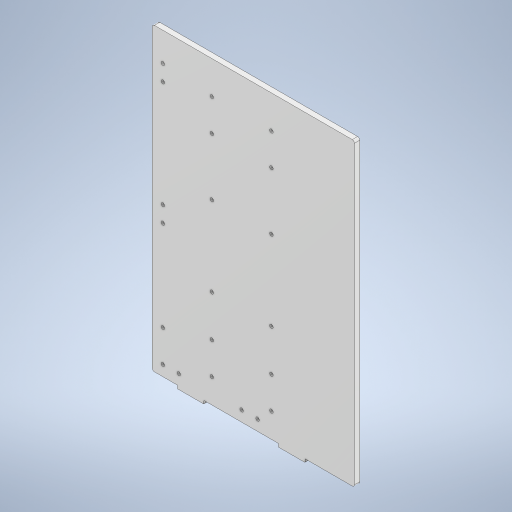
# Autodesk Inventor part: BP_Exterior-Right-Ver2
Saved by Autodesk Inventor 2024.3 (Build 283343000, 343)
## iProperties
Created: 2025-04-22
Part Number: BP_Exterior-Right-Ver2
Material: PBT プラスチック
Document SubType Name: Modeling
Designer: ngt-a
Density: 1.31 g/cm^3
Appearance: 滑らか - 白
Mass: 278.324 g
Surface Area: 1185.79 cm^2
Volume: 212.461 cm^3
Author: ngt-a
Autodesk Inventor part; units mm, degrees
ref_plane "YZ Plane" through (0, 0, 0) normal (1, 0, 0) x (0, 1, 0)
ref_plane "XZ Plane" through (0, 0, 0) normal (0, 1, 0) x (-1, 0, 0)
ref_plane "XY Plane" through (0, 0, 0) normal (0, 0, 1) x (1, 0, 0)
sketch "スケッチ22" plane through (0, 0, 0) normal (0, 0, 1) x (1, 0, 0)
  line L0 (0, 0) -> (190, 0)
  line L1 (190, 0) -> (190, 305)
  line L2 (190, 305) -> (0, 305)
  line L3 (0, 305) -> (0, 0)
  dimension "d163" = 190
  dimension "d164" = 305
  constraints: 8 end point, 2 parallel, 1 horizontal, 1 perpendicular
  measures "d163" distance of L1.end L2.end
  measures "d164" distance of L0.end L1.end
extrude "押し出し20" add sketch "スケッチ22" along normal blind 3
sketch "スケッチ23" plane through (0, 0, 3) normal (0, 0, 1) x (1, 0, 0)
  line L0 (0, 0) -> (190, 0) projected
  line L1 (190, 0) -> (190, 305) projected
  line L2 (0, 305) -> (0, 0) projected
  line L3 (190, 305) -> (0, 305) projected
  point P0 (134, 26)
  point P1 (78, 26)
  point P2 (78, 56)
  point P3 (134, 56)
  point P4 (78, 224)
  point P5 (134, 224)
  point P6 (134, 254)
  point P7 (78, 254)
  point P8 (134, 95)
  point P9 (134, 170)
  point P10 (78, 170)
  point P11 (78, 95)
  dimension "d167" = 56
  dimension "d168" = 30
  dimension "d169" = 30
  dimension "d170" = 56
  dimension "d171" = 56
  dimension "d172" = 56
  dimension "d173" = 30
  dimension "d174" = 30
  dimension "d175" = 75
  dimension "d176" = 75
  dimension "d177" = 56
  dimension "d178" = 56
  dimension "d179" = 26
  dimension "d180" = 26
  dimension "d181" = 39
  dimension "d182" = 39
  dimension "d183" = 54
  dimension "d184" = 54
  dimension "d185" = 56
  dimension "d316" = 56
  dimension "d317" = 56
  dimension "d318" = 78
  dimension "d319" = 51
  measures "d167" distance of point (134, 56) point (78, 56)
  measures "d168" distance of point (134, 26) point (134, 56)
  measures "d169" distance of point (78, 56) point (78, 26)
  measures "d170" distance of point (134, 26) point (78, 26)
  measures "d171" distance of point (134, 224) point (78, 224)
  measures "d172" distance of point (134, 254) point (78, 254)
  measures "d173" distance of point (134, 224) point (134, 254)
  measures "d174" distance of point (78, 254) point (78, 224)
  measures "d175" distance of point (134, 95) point (134, 170)
  measures "d176" distance of point (78, 170) point (78, 95)
  measures "d177" distance of point (134, 95) point (78, 95)
  measures "d178" distance of point (134, 170) point (78, 170)
  measures "d179" distance from line of L0 point (134, 26)
  measures "d180" distance from line of L0 point (78, 26)
  measures "d181" distance of point (134, 56) point (134, 95)
  measures "d182" distance of point (78, 56) point (78, 95)
  measures "d183" distance of point (134, 170) point (134, 224)
  measures "d184" distance of point (78, 170) point (78, 224)
  measures "d185" distance from line of L1 point (134, 26)
  measures "d316" distance from line of L1 point (134, 224)
  measures "d317" distance from line of L1 point (134, 254)
  measures "d318" distance from line of L2 point (78, 254)
  measures "d319" distance from line of L3 point (78, 254)
hole "穴2" at (134, 26, 3) at (78, 26, 3) at (78, 56, 3) at (134, 56, 3) at (78, 224, 3) at (134, 224, 3) at (134, 254, 3) at (78, 254, 3) at (134, 95, 3) at (134, 170, 3) at (78, 170, 3) at (78, 95, 3) direction (0, 0, -1) diameter 3.2 end through all
sketch "スケッチ24" plane through (0, 0, 3) normal (0, 0, 1) x (1, 0, 0)
  line L0 (0, 305) -> (0, 0) projected
  line L1 (0, 0) -> (190, 0) projected
  line L2 (190, 0) -> (190, 305) projected
  point P0 (91, 13)
  point P1 (106, 13)
  point P2 (165, 13)
  point P3 (180, 13)
  dimension "d193" = 15
  dimension "d195" = 13
  dimension "d196" = 13
  dimension "d204" = 15
  dimension "d205" = 13
  dimension "d207" = 13
  dimension "d217" = 59
  dimension "d219" = 10
  measures "d193" distance of point (106, 13) point (91, 13)
  measures "d195" distance from line of L1 point (106, 13)
  measures "d196" distance from line of L1 point (91, 13)
  measures "d204" distance of point (165, 13) point (180, 13)
  measures "d205" distance from line of L1 point (165, 13)
  measures "d207" distance from line of L1 point (180, 13)
  measures "d217" distance of point (106, 13) point (165, 13)
  measures "d219" distance from line of L2 point (180, 13)
hole "穴3" at (91, 13, 3) at (106, 13, 3) at (165, 13, 3) at (180, 13, 3) direction (0, 0, -1) diameter 3.2 end through all
sketch "スケッチ25" plane through (0, 0, 3) normal (0, 0, 1) x (1, 0, 0)
  line L0 (0, 0) -> (46.3, 0)
  line L1 (46.3, 0) -> (46.3, 3)
  line L2 (46.3, 3) -> (0, 3)
  line L3 (0, 3) -> (0, 0)
  line L4 (71.5, 0) -> (141.3, 0)
  line L5 (141.3, 0) -> (141.3, 3)
  line L6 (141.3, 3) -> (71.5, 3)
  line L7 (71.5, 3) -> (71.5, 0)
  line L8 (190, 0) -> (190, 305) projected
  line L9 (190, 0) -> (166.5, 0)
  line L10 (166.5, 0) -> (166.5, 3)
  line L11 (166.5, 3) -> (190, 3)
  line L12 (190, 3) -> (190, 0)
  point P0 (46.3, 1.5)
  point P1 (71.5, 1.5)
  point P2 (166.5, 1.5)
  point P3 (141.3, 1.5)
  point P4 (190, 1.5)
  dimension "d209" = 3
  dimension "d210" = 3
  dimension "d211" = 3
  dimension "d212" = 25.2
  dimension "d213" = 25.2
  dimension "d221" = 23.5
  dimension "d222" = 69.8
  constraints: 24 end point, 6 parallel, 5 midpoint, 3 horizontal, 3 perpendicular, 1 point on line
  measures "d209" distance of L0.end L1.end
  measures "d210" distance between parallel lines of L4 L6
  measures "d211" distance between parallel lines of L9 L11
  measures "d212" distance of point (46.3, 1.5) point (71.5, 1.5)
  measures "d213" distance of point (166.5, 1.5) point (141.3, 1.5)
  measures "d221" distance of point (190, 1.5) point (166.5, 1.5)
  measures "d222" distance of L5.end L6.end
extrude "押し出し21" cut sketch "スケッチ25" against normal through all
sketch "スケッチ26" plane through (0, 0, 0) normal (0, 0, -1) x (-1, 0, 0)
  line L0 (-190, 305) -> (0, 305) projected
  line L1 (0, 305) -> (0, 3) projected
  line L2 (-190, 305) -> (0, 305)
  line L3 (0, 305) -> (0, 285)
  line L4 (0, 285) -> (-190, 285)
  line L5 (-190, 285) -> (-190, 305)
  line L6 (0, 305) -> (-10, 305)
  line L7 (-10, 305) -> (-10, 0)
  line L8 (-10, 0) -> (0, 0)
  line L9 (0, 0) -> (0, 305)
  line L10 (-141.3, 0) -> (-166.5, 0) projected
  line L11 (-190, 3) -> (-190, 305) projected
  point P0 (0, 0)
  point P1 (-10, 285)
  dimension "d223" = 20
  dimension "d228" = 305
  dimension "d229" = 190
  constraints: 16 end point, 4 parallel, 2 horizontal, 2 perpendicular, 1 point on line
  measures "d223" distance between parallel lines of L0 L4
  measures "d228" distance between parallel lines of L10 L0
  measures "d229" distance between parallel lines of L1 L11
extrude "押し出し22" cut sketch "スケッチ26" against normal blind 10 contours L0 L7 L4 L5 | L0 L1 L4 L7
fillet "フィレット2" radius 2 4 edges at (190, 285, 1.5) (190, 3, 1.5) (0, 3, 1.5) (0, 285, 1.5)
sketch "スケッチ27" plane through (141.3, 0, 0) normal (0, -1, 0) x (1, 0, 0)
  line L0 (-95, 3) -> (-69.8, 3) projected
  line L1 (-69.8, 3) -> (-95, 3)
  line L2 (-95, 3) -> (-95, 0)
  line L3 (-95, 0) -> (-69.8, 0)
  line L4 (-69.8, 0) -> (-69.8, 3)
  line L5 (25.2, 3) -> (25.2, 0) projected
  line L6 (25.2, 3) -> (0, 3)
  line L7 (0, 3) -> (0, 0)
  line L8 (0, 0) -> (25.2, 0)
  line L9 (25.2, 0) -> (25.2, 3)
  line L10 (-69.9, 0.1) -> (-94.9, 0.1)
  line L11 (-94.9, 0.1) -> (-94.9, 2.9)
  line L12 (-94.9, 2.9) -> (-69.9, 2.9)
  line L13 (-69.9, 2.9) -> (-69.9, 0.1)
  line L14 (25.1, 0.1) -> (0.1, 0.1)
  line L15 (0.1, 0.1) -> (0.1, 2.9)
  line L16 (0.1, 2.9) -> (25.1, 2.9)
  line L17 (25.1, 2.9) -> (25.1, 0.1)
  line L18 (-69.8, 3) -> (-69.9, 3)
  line L19 (-69.9, 3) -> (-69.9, 0)
  line L20 (-69.9, 0) -> (-69.8, 0)
  line L21 (-69.8, 0) -> (-69.8, 3)
  line L22 (-95, 3) -> (-94.9, 3)
  line L23 (-94.9, 3) -> (-94.9, 0)
  line L24 (-94.9, 0) -> (-95, 0)
  line L25 (-95, 0) -> (-95, 3)
  line L26 (0, 3) -> (0.1, 3)
  line L27 (0.1, 3) -> (0.1, 0)
  line L28 (0.1, 0) -> (0, 0)
  line L29 (0, 0) -> (0, 3)
  line L30 (25.2, 3) -> (25.1, 3)
  line L31 (25.1, 3) -> (25.1, 0)
  line L32 (25.1, 0) -> (25.2, 0)
  line L33 (25.2, 0) -> (25.2, 3)
  point P0 (-141.3, 0)
  point P1 (-69.8, 1.5)
  point P2 (-95, 1.5)
  point P3 (0.1, 2.9)
  point P4 (0.1, 3)
  point P5 (0.1, 0.1)
  point P6 (25.1, 0.1)
  point P7 (25.1, 3)
  point P8 (25.1, 2.9)
  dimension "d231" = 3
  dimension "d232" = 25.2
  dimension "d233" = 0.1
  dimension "d234" = 0.1
  constraints: 64 end point, 16 parallel, 8 perpendicular, 6 horizontal, 6 point on line, 2 midpoint, 6 other
  measures "d231" distance between parallel lines of L0 L3
  measures "d232" distance of point (-69.8, 1.5) point (-95, 1.5)
  measures "d233" distance between parallel lines of L8 L14
  measures "d234" distance between parallel lines of L3 L10
extrude "押し出し23" cut sketch "スケッチ27" against normal blind 3 contours L0 L23 L11 L3 L2 | L0 L4 L3 L19 L13 | L5 L8 L31 L17 L6 | L27 L15 L8 L7 L6
sketch "スケッチ28" plane through (0, 0, 0) normal (0, 0, -1) x (-1, 0, 0)
  line L0 (-71.4, 3) -> (-71.4, 0) projected
  line L1 (-46.4, 0) -> (-71.4, 0) projected
  line L2 (-46.4, 0) -> (-46.4, 3) projected
  line L3 (-46.4, 3) -> (-2, 3) projected
  arc A0 (-2, 3) -> (0, 5) centre (-2, 5) ccw projected
  line L4 (0, 283) -> (0, 5) projected
  arc A1 (0, 283) -> (-2, 285) centre (-2, 283) ccw projected
  line L5 (-2, 285) -> (-188, 285) projected
  arc A2 (-188, 285) -> (-190, 283) centre (-188, 283) ccw projected
  line L6 (-190, 5) -> (-190, 283) projected
  arc A3 (-190, 5) -> (-188, 3) centre (-188, 5) ccw projected
  line L7 (-188, 3) -> (-166.4, 3) projected
  line L8 (-166.4, 3) -> (-166.4, 0) projected
  line L9 (-141.4, 0) -> (-166.4, 0) projected
  line L10 (-141.4, 0) -> (-141.4, 3) projected
  line L11 (-141.4, 3) -> (-71.4, 3) projected
  circle A4 centre (-134, 26) radius 1.6 projected
  circle A5 centre (-78, 26) radius 1.6 projected
  circle A6 centre (-78, 56) radius 1.6 projected
  circle A7 centre (-134, 56) radius 1.6 projected
  circle A8 centre (-78, 224) radius 1.6 projected
  circle A9 centre (-134, 224) radius 1.6 projected
  circle A10 centre (-134, 254) radius 1.6 projected
  circle A11 centre (-78, 254) radius 1.6 projected
  circle A12 centre (-134, 95) radius 1.6 projected
  circle A13 centre (-134, 170) radius 1.6 projected
  circle A14 centre (-78, 170) radius 1.6 projected
  circle A15 centre (-78, 95) radius 1.6 projected
  circle A16 centre (-91, 13) radius 1.6 projected
  circle A17 centre (-106, 13) radius 1.6 projected
  circle A18 centre (-165, 13) radius 1.6 projected
  circle A19 centre (-180, 13) radius 1.6 projected
  line L12 (-190, 285) -> (0, 285)
  line L13 (0, 285) -> (0, 3)
  line L14 (0, 3) -> (-190, 3)
  line L15 (-190, 3) -> (-190, 285)
  point P0 (0, 0)
  constraints: 8 end point, 2 parallel, 2 point on line, 1 horizontal, 1 perpendicular
extrude "押し出し24" add sketch "スケッチ28" along normal blind 2 contours L11 L14 L7 A3 L6 A2 L5 A1 L4 A0 L3
sketch "スケッチ29" plane through (0, 0, -2) normal (0, 0, -1) x (-1, 0, 0)
  line L0 (-188, 3) -> (-2, 3) projected
  arc A0 (-2, 3) -> (0, 5) centre (-2, 5) ccw projected
  line L1 (0, 5) -> (0, 283) projected
  arc A1 (0, 283) -> (-2, 285) centre (-2, 283) ccw projected
  line L2 (-2, 285) -> (-188, 285) projected
  arc A2 (-188, 285) -> (-190, 283) centre (-188, 283) ccw projected
  line L3 (-190, 283) -> (-190, 5) projected
  arc A3 (-190, 5) -> (-188, 3) centre (-188, 5) ccw projected
  circle A4 centre (-165, 13) radius 1.6 projected
  circle A5 centre (-91, 13) radius 1.6 projected
  circle A6 centre (-78, 170) radius 1.6 projected
  circle A7 centre (-134, 95) radius 1.6 projected
  circle A8 centre (-134, 254) radius 1.6 projected
  circle A9 centre (-134, 26) radius 1.6 projected
  circle A10 centre (-78, 26) radius 1.6 projected
  circle A11 centre (-78, 56) radius 1.6 projected
  circle A12 centre (-134, 56) radius 1.6 projected
  circle A13 centre (-78, 224) radius 1.6 projected
  circle A14 centre (-134, 224) radius 1.6 projected
  circle A15 centre (-78, 254) radius 1.6 projected
  circle A16 centre (-134, 170) radius 1.6 projected
  circle A17 centre (-78, 95) radius 1.6 projected
  circle A18 centre (-106, 13) radius 1.6 projected
  circle A19 centre (-180, 13) radius 1.6 projected
  line L4 (-190, 20) -> (0, 20)
  line L5 (-46.4, 0) -> (-71.4, 0) projected
  circle A20 centre (-134, 26) radius 3.75
  circle A21 centre (-78, 26) radius 3.75
  circle A22 centre (-134, 56) radius 3.75
  circle A23 centre (-78, 56) radius 3.75
  circle A24 centre (-134, 95) radius 3.75
  circle A25 centre (-78, 95) radius 3.75
  circle A26 centre (-134, 170) radius 3.75
  circle A27 centre (-78, 170) radius 3.75
  circle A28 centre (-134, 224) radius 3.75
  circle A29 centre (-78, 224) radius 3.75
  circle A30 centre (-134, 254) radius 3.75
  circle A31 centre (-78, 254) radius 3.75
  line L6 (-20, 285) -> (-20, 3)
  line L7 (-111.1, 20) -> (-85.9, 20)
  line L8 (-85.9, 20) -> (-85.9, 30)
  line L9 (-85.9, 30) -> (-111.1, 30)
  line L10 (-111.1, 30) -> (-111.1, 20)
  line L11 (-159.9, 20) -> (-185.1, 20)
  line L12 (-185.1, 20) -> (-185.1, 30)
  line L13 (-185.1, 30) -> (-159.9, 30)
  line L14 (-159.9, 30) -> (-159.9, 20)
  point P0 (0, 0)
  point P1 (-185.1, 25)
  point P2 (-98.5, 30)
  point P3 (-111.1, 25)
  point P4 (-20, 20)
  point P5 (-85.9, 20)
  dimension "d239" = 20
  dimension "d242" = 7.5
  dimension "d243" = 7.5
  dimension "d244" = 7.5
  dimension "d245" = 7.5
  dimension "d246" = 7.5
  dimension "d247" = 7.5
  dimension "d248" = 7.5
  dimension "d249" = 7.5
  dimension "d250" = 7.5
  dimension "d251" = 7.5
  dimension "d252" = 7.5
  dimension "d253" = 7.5
  dimension "d254" = 20
  dimension "d256" = 5.1
  dimension "d257" = 10
  dimension "d258" = 10
  dimension "d259" = 5.1
  dimension "d263" = 5.1
  dimension "d264" = 5.1
  constraints: 20 end point, 12 centre point, 6 point on line, 4 parallel, 4 perpendicular, 3 midpoint, 2 horizontal
  measures "d239" distance between parallel lines of L5 L4
  measures "d242" diameter of A30
  measures "d243" diameter of A31
  measures "d244" diameter of A28
  measures "d245" diameter of A29
  measures "d246" diameter of A26
  measures "d247" diameter of A27
  measures "d248" diameter of A24
  measures "d249" diameter of A25
  measures "d250" diameter of A22
  measures "d251" diameter of A23
  measures "d252" diameter of A20
  measures "d253" diameter of A21
  measures "d254" distance between parallel lines of L1 L6
  measures "d256" horizontal distance of A19.centre point (-185.1, 25)
  measures "d257" distance between parallel lines of L4 L13
  measures "d258" distance from line of L7 point (-98.5, 30)
  measures "d259" distance from line of A18.centre L10
  measures "d263" distance from line of A4.centre L14
  measures "d264" distance from line of A5.centre L8
extrude "押し出し25" cut sketch "スケッチ29" against normal blind 2 contours A3 L3 L4 L6 L0 | L4 L10 L9 L8 | L12 L13 L14 L4 | A6 | A7 | A8 | A9 | A12 | A13 | A14 | A15 | A16 | A17 | A20 | A21 | A22 | A23 | A24 | A25 | A26 | A27 | A28 | A29 | A30 | A31
fillet "フィレット3" radius 2 11 edges at (190, 20, -1) (185.1, 20, -1) (185.1, 30, -1) (159.9, 30, -1) (159.9, 20, -1) (111.1, 20, -1) (111.1, 30, -1) (85.9, 30, -1) (85.9, 20, -1) (20, 20, -1) (20, 3, -1)
fillet "フィレット4" radius 0.2 8 edges at (166.4, 3, 1.5) (166.4, 0, 1.5) (141.4, 0, 1.5) (141.4, 3, 1.5) (71.4, 0, 1.5) (46.4, 0, 1.5) (46.4, 3, 1.5) (71.4, 3, 1.5)
sketch "スケッチ31" plane through (0, 0, -2) normal (0, 0, -1) x (-1, 0, 0)
  circle A0 centre (-180, 13) radius 1.6 projected
  line L0 (-190, 283) -> (-190, 22) projected
  point P0 (0, 0)
  point P1 (-180, 43)
  point P2 (-180, 128)
  point P3 (-180, 258)
  point P4 (-180, 143)
  point P5 (-180, 243)
  dimension "d265" = 30
  dimension "d266" = 10
  dimension "d267" = 10
  dimension "d268" = 85
  dimension "d269" = 15
  dimension "d270" = 100
  dimension "d271" = 15
  dimension "d272" = 10
  dimension "d273" = 10
  dimension "d274" = 10
  measures "d265" distance of A0.centre point (-180, 43)
  measures "d266" distance from line of L0 point (-180, 43)
  measures "d267" distance from line of L0 point (-180, 128)
  measures "d268" distance of point (-180, 43) point (-180, 128)
  measures "d269" distance of point (-180, 128) point (-180, 143)
  measures "d270" distance of point (-180, 143) point (-180, 243)
  measures "d271" distance of point (-180, 243) point (-180, 258)
  measures "d272" distance from line of L0 point (-180, 143)
  measures "d273" distance from line of L0 point (-180, 243)
  measures "d274" distance from line of L0 point (-180, 258)
hole "穴4" at (180, 43, -2) at (180, 128, -2) at (180, 258, -2) at (180, 143, -2) at (180, 243, -2) direction (0, 0, 1) diameter 3.2 depth 61.5 tip angle 118
sketch "スケッチ32" plane through (0, 0, -2) normal (0, 0, -1) x (-1, 0, 0)
  arc A0 (-46.6, 0) -> (-46.4, 0.2) centre (-46.6, 0.2) ccw projected
  line L0 (-46.4, 0.2) -> (-46.4, 2.8) projected
  arc A1 (-46.2, 3) -> (-46.4, 2.8) centre (-46.2, 2.8) ccw projected
  line L1 (-18, 3) -> (-46.2, 3) projected
  arc A2 (-20, 5) -> (-18, 3) centre (-18, 5) ccw projected
  line L2 (-20, 18) -> (-20, 5) projected
  arc A3 (-20, 18) -> (-22, 20) centre (-22, 18) ccw projected
  line L3 (-83.9, 20) -> (-22, 20) projected
  arc A4 (-85.9, 22) -> (-83.9, 20) centre (-83.9, 22) ccw projected
  line L4 (-85.9, 28) -> (-85.9, 22) projected
  arc A5 (-85.9, 28) -> (-87.9, 30) centre (-87.9, 28) ccw projected
  line L5 (-109.1, 30) -> (-87.9, 30) projected
  arc A6 (-109.1, 30) -> (-111.1, 28) centre (-109.1, 28) ccw projected
  line L6 (-111.1, 22) -> (-111.1, 28) projected
  arc A7 (-113.1, 20) -> (-111.1, 22) centre (-113.1, 22) ccw projected
  line L7 (-157.9, 20) -> (-113.1, 20) projected
  arc A8 (-159.9, 22) -> (-157.9, 20) centre (-157.9, 22) ccw projected
  line L8 (-159.9, 28) -> (-159.9, 22) projected
  arc A9 (-159.9, 28) -> (-161.9, 30) centre (-161.9, 28) ccw projected
  line L9 (-183.1, 30) -> (-161.9, 30) projected
  arc A10 (-183.1, 30) -> (-185.1, 28) centre (-183.1, 28) ccw projected
  line L10 (-185.1, 22) -> (-185.1, 28) projected
  arc A11 (-187.1, 20) -> (-185.1, 22) centre (-187.1, 22) ccw projected
  line L11 (-188, 20) -> (-187.1, 20) projected
  arc A12 (-190, 22) -> (-188, 20) centre (-188, 22) ccw projected
  line L12 (-190, 5) -> (-190, 22) projected
  arc A13 (-190, 5) -> (-188, 3) centre (-188, 5) ccw projected
  line L13 (-166.6, 3) -> (-188, 3) projected
  arc A14 (-166.4, 2.8) -> (-166.6, 3) centre (-166.6, 2.8) ccw projected
  line L14 (-166.4, 2.8) -> (-166.4, 0.2) projected
  arc A15 (-166.4, 0.2) -> (-166.2, 0) centre (-166.2, 0.2) ccw projected
  line L15 (-141.6, 0) -> (-166.2, 0) projected
  arc A16 (-141.6, 0) -> (-141.4, 0.2) centre (-141.6, 0.2) ccw projected
  line L16 (-141.4, 0.2) -> (-141.4, 2.8) projected
  arc A17 (-141.2, 3) -> (-141.4, 2.8) centre (-141.2, 2.8) ccw projected
  line L17 (-71.6, 3) -> (-141.2, 3) projected
  arc A18 (-71.4, 2.8) -> (-71.6, 3) centre (-71.6, 2.8) ccw projected
  line L18 (-71.4, 2.8) -> (-71.4, 0.2) projected
  arc A19 (-71.4, 0.2) -> (-71.2, 0) centre (-71.2, 0.2) ccw projected
  line L19 (-46.6, 0) -> (-71.2, 0) projected
  circle A20 centre (-180, 13) radius 1.6 projected
  circle A21 centre (-106, 13) radius 1.6 projected
  circle A22 centre (-91, 13) radius 1.6 projected
  circle A23 centre (-165, 13) radius 1.6 projected
  circle A24 centre (-180, 243) radius 1.6 projected
  circle A25 centre (-180, 143) radius 1.6 projected
  circle A26 centre (-180, 258) radius 1.6 projected
  circle A27 centre (-180, 128) radius 1.6 projected
  arc A28 (-20, 5) -> (-18, 3) centre (-18, 5) ccw projected
  line L20 (-18, 3) -> (-2, 3) projected
  arc A29 (-2, 3) -> (0, 5) centre (-2, 5) ccw projected
  line L21 (0, 5) -> (0, 283) projected
  arc A30 (0, 283) -> (-2, 285) centre (-2, 283) ccw projected
  line L22 (-2, 285) -> (-188, 285) projected
  arc A31 (-188, 285) -> (-190, 283) centre (-188, 283) ccw projected
  line L23 (-190, 283) -> (-190, 22) projected
  arc A32 (-190, 22) -> (-188, 20) centre (-188, 22) ccw projected
  line L24 (-188, 20) -> (-187.1, 20) projected
  arc A33 (-187.1, 20) -> (-185.1, 22) centre (-187.1, 22) ccw projected
  line L25 (-185.1, 22) -> (-185.1, 28) projected
  arc A34 (-183.1, 30) -> (-185.1, 28) centre (-183.1, 28) ccw projected
  line L26 (-183.1, 30) -> (-161.9, 30) projected
  arc A35 (-159.9, 28) -> (-161.9, 30) centre (-161.9, 28) ccw projected
  line L27 (-159.9, 28) -> (-159.9, 22) projected
  arc A36 (-159.9, 22) -> (-157.9, 20) centre (-157.9, 22) ccw projected
  line L28 (-157.9, 20) -> (-113.1, 20) projected
  arc A37 (-113.1, 20) -> (-111.1, 22) centre (-113.1, 22) ccw projected
  line L29 (-111.1, 22) -> (-111.1, 28) projected
  arc A38 (-109.1, 30) -> (-111.1, 28) centre (-109.1, 28) ccw projected
  line L30 (-109.1, 30) -> (-87.9, 30) projected
  arc A39 (-85.9, 28) -> (-87.9, 30) centre (-87.9, 28) ccw projected
  line L31 (-85.9, 28) -> (-85.9, 22) projected
  arc A40 (-85.9, 22) -> (-83.9, 20) centre (-83.9, 22) ccw projected
  line L32 (-83.9, 20) -> (-22, 20) projected
  arc A41 (-20, 18) -> (-22, 20) centre (-22, 18) ccw projected
  line L33 (-20, 18) -> (-20, 5) projected
  circle A42 centre (-78, 26) radius 3.75 projected
  circle A43 centre (-78, 170) radius 3.75 projected
  circle A44 centre (-78, 254) radius 3.75 projected
  circle A45 centre (-134, 224) radius 3.75 projected
  circle A46 centre (-134, 95) radius 3.75 projected
  circle A47 centre (-134, 26) radius 3.75 projected
  circle A48 centre (-78, 56) radius 3.75 projected
  circle A49 centre (-134, 170) radius 3.75 projected
  circle A50 centre (-134, 254) radius 3.75 projected
  circle A51 centre (-78, 224) radius 3.75 projected
  circle A52 centre (-78, 95) radius 3.75 projected
  circle A53 centre (-134, 56) radius 3.75 projected
  circle A54 centre (-180, 128) radius 3.75
  circle A55 centre (-180, 143) radius 3.75
  circle A56 centre (-180, 243) radius 3.75
  circle A57 centre (-180, 258) radius 3.75
  circle A58 centre (-180, 243) radius 1.6 projected
  circle A59 centre (-180, 143) radius 1.6 projected
  circle A60 centre (-180, 258) radius 1.6 projected
  circle A61 centre (-180, 128) radius 1.6 projected
  circle A62 centre (-180, 43) radius 1.6 projected
  arc A63 (-20, 5) -> (-18, 3) centre (-18, 5) ccw projected
  line L34 (-18, 3) -> (-2, 3) projected
  arc A64 (-2, 3) -> (0, 5) centre (-2, 5) ccw projected
  line L35 (0, 5) -> (0, 283) projected
  arc A65 (0, 283) -> (-2, 285) centre (-2, 283) ccw projected
  line L36 (-2, 285) -> (-188, 285) projected
  arc A66 (-188, 285) -> (-190, 283) centre (-188, 283) ccw projected
  line L37 (-190, 283) -> (-190, 22) projected
  arc A67 (-190, 22) -> (-188, 20) centre (-188, 22) ccw projected
  line L38 (-188, 20) -> (-187.1, 20) projected
  arc A68 (-187.1, 20) -> (-185.1, 22) centre (-187.1, 22) ccw projected
  line L39 (-185.1, 22) -> (-185.1, 28) projected
  arc A69 (-183.1, 30) -> (-185.1, 28) centre (-183.1, 28) ccw projected
  line L40 (-183.1, 30) -> (-161.9, 30) projected
  arc A70 (-159.9, 28) -> (-161.9, 30) centre (-161.9, 28) ccw projected
  line L41 (-159.9, 28) -> (-159.9, 22) projected
  arc A71 (-159.9, 22) -> (-157.9, 20) centre (-157.9, 22) ccw projected
  line L42 (-157.9, 20) -> (-113.1, 20) projected
  arc A72 (-113.1, 20) -> (-111.1, 22) centre (-113.1, 22) ccw projected
  line L43 (-111.1, 22) -> (-111.1, 28) projected
  arc A73 (-109.1, 30) -> (-111.1, 28) centre (-109.1, 28) ccw projected
  line L44 (-109.1, 30) -> (-87.9, 30) projected
  arc A74 (-85.9, 28) -> (-87.9, 30) centre (-87.9, 28) ccw projected
  line L45 (-85.9, 28) -> (-85.9, 22) projected
  arc A75 (-85.9, 22) -> (-83.9, 20) centre (-83.9, 22) ccw projected
  line L46 (-83.9, 20) -> (-22, 20) projected
  arc A76 (-20, 18) -> (-22, 20) centre (-22, 18) ccw projected
  line L47 (-20, 18) -> (-20, 5) projected
  circle A77 centre (-78, 26) radius 3.75 projected
  circle A78 centre (-78, 170) radius 3.75 projected
  circle A79 centre (-78, 254) radius 3.75 projected
  circle A80 centre (-134, 224) radius 3.75 projected
  circle A81 centre (-134, 95) radius 3.75 projected
  circle A82 centre (-134, 26) radius 3.75 projected
  circle A83 centre (-78, 56) radius 3.75 projected
  circle A84 centre (-134, 170) radius 3.75 projected
  circle A85 centre (-134, 254) radius 3.75 projected
  circle A86 centre (-78, 224) radius 3.75 projected
  circle A87 centre (-78, 95) radius 3.75 projected
  circle A88 centre (-134, 56) radius 3.75 projected
  circle A89 centre (-180, 43) radius 3.75
  point P0 (0, 0)
  dimension "d282" = 7.5
  dimension "d283" = 7.5
  dimension "d284" = 7.5
  dimension "d285" = 7.5
  dimension "d289" = 7.5
  constraints: 5 centre point
  measures "d282" diameter of A57
  measures "d283" diameter of A56
  measures "d284" diameter of A55
  measures "d285" diameter of A54
  measures "d289" diameter of A89
extrude "押し出し26" cut sketch "スケッチ32" against normal blind 2 contours A24 | A25 | A26 | A27 | A54 | A55 | A56 | A57 | A89
sketch "スケッチ34" plane through (0, 0, -2) normal (0, 0, -1) x (-1, 0, 0)
  circle A0 centre (-134, 56) radius 1.6 projected
  circle A1 centre (-78, 26) radius 1.6 projected
  line L0 (-134, 56) -> (-78, 26)
  circle A2 centre (-134, 26) radius 1.6 projected
  line L1 (-78, 26) -> (-134, 26)
  circle A3 centre (-78, 56) radius 1.6 projected
  line L2 (-134, 26) -> (-78, 56)
  line L3 (-78, 56) -> (-134, 56)
  line L4 (-134, 26) -> (-134, 56)
  line L5 (-78, 26) -> (-78, 56)
  circle A4 centre (-134, 95) radius 1.6 projected
  line L6 (-134, 95) -> (-78, 95)
  circle A5 centre (-78, 170) radius 1.6 projected
  line L7 (-78, 95) -> (-78, 170)
  circle A6 centre (-134, 170) radius 1.6 projected
  line L8 (-78, 170) -> (-134, 170)
  line L9 (-134, 170) -> (-134, 95)
  circle A7 centre (-78, 170) radius 3.75 projected
  line L10 (-78, 170) -> (-134, 95)
  line L11 (-78, 95) -> (-134, 170)
  circle A8 centre (-134, 224) radius 1.6 projected
  circle A9 centre (-134, 254) radius 1.6 projected
  line L12 (-134, 224) -> (-134, 254)
  circle A10 centre (-78, 254) radius 1.6 projected
  line L13 (-134, 254) -> (-78, 254)
  circle A11 centre (-78, 224) radius 1.6 projected
  line L14 (-78, 254) -> (-78, 224)
  line L15 (-78, 224) -> (-134, 224)
  line L16 (-78, 254) -> (-134, 224)
  line L17 (-134, 254) -> (-78, 224)
  line L18 (-134, 251) -> (-78, 251)
  line L19 (-132.5833, 256.6444) -> (-76.5833, 226.6444)
  line L20 (-79.4167, 256.6444) -> (-135.4167, 226.6444)
  line L21 (-131, 224) -> (-131, 254)
  line L22 (-135.4167, 251.3556) -> (-79.4167, 221.3556)
  line L23 (-78, 227) -> (-134, 227)
  line L24 (-76.5833, 251.3556) -> (-132.5833, 221.3556)
  line L25 (-81, 254) -> (-81, 224)
  line L26 (-134, 167) -> (-81, 167)
  line L27 (-81, 167) -> (-81, 95)
  line L28 (-131, 170) -> (-131, 95)
  line L29 (-134, 98) -> (-78, 98)
  line L30 (-75.5962, 168.2051) -> (-131.5962, 93.2051)
  line L31 (-80.4038, 93.2051) -> (-136.4038, 168.2051)
  line L32 (-80.4038, 171.7949) -> (-136.4038, 96.7949)
  line L33 (-75.5962, 96.7949) -> (-131.5962, 171.7949)
  line L34 (-78, 53) -> (-134, 53)
  line L35 (-132.5833, 58.6444) -> (-66.047, 23)
  line L36 (-66.047, 23) -> (-134, 23)
  line L37 (-81, 26) -> (-81, 56)
  line L38 (-132.5833, 23.3556) -> (-76.5833, 53.3556)
  line L39 (-135.4167, 53.3556) -> (-89.953, 29)
  line L40 (-89.953, 29) -> (-134, 29)
  line L41 (-131, 26) -> (-131, 56)
  line L42 (-135.4167, 28.6444) -> (-79.4167, 58.6444)
  circle A12 centre (-134, 224) radius 3.75 projected
  line L43 (-134, 224) -> (-134, 170)
  line L44 (-78, 224) -> (-78, 170)
  line L45 (-134, 95) -> (-134, 56)
  circle A13 centre (-78, 95) radius 1.6 projected
  line L46 (-78, 95) -> (-78, 56)
  line L47 (-134, 56) -> (-78, 95)
  line L48 (-134, 95) -> (-78, 56)
  line L49 (-134, 170) -> (-78, 224)
  line L50 (-134, 224) -> (-78, 170)
  line L51 (-78, 221) -> (-134, 221)
  line L52 (-131, 170) -> (-131, 216.9396)
  line L53 (-131, 216.9396) -> (-80.0824, 167.8405)
  line L54 (-75.9176, 172.1595) -> (-137, 231.0604)
  line L55 (-137, 231.0604) -> (-137, 170)
  line L56 (-136.0824, 172.1595) -> (-80.0824, 226.1595)
  line L57 (-131.9176, 167.8405) -> (-75.9176, 221.8405)
  line L58 (-134, 173) -> (-75, 173)
  line L59 (-75, 173) -> (-75, 95)
  line L60 (-81, 224) -> (-81, 170)
  line L61 (-134, 92) -> (-78, 92)
  line L62 (-131, 95) -> (-131, 56)
  line L63 (-81, 56) -> (-81, 89.2549)
  line L64 (-81, 89.2549) -> (-132.2855, 53.5382)
  line L65 (-132.2855, 97.4618) -> (-76.2855, 58.4618)
  line L66 (-135.7145, 58.4618) -> (-75, 100.7451)
  line L67 (-75, 100.7451) -> (-75, 56)
  line L68 (-78, 59) -> (-134, 59)
  line L69 (-135.7145, 92.5382) -> (-79.7145, 53.5382)
  point P0 (0, 0)
  point P1 (-131, 239)
  point P2 (-131, 41)
  point P3 (-81, 229.0105)
  point P4 (-81, 248.9895)
  point P5 (-99.647, 239)
  point P6 (-106, 235.5966)
  point P7 (-122.047, 227)
  point P8 (-89.953, 227)
  point P9 (-112.353, 239)
  point P10 (-131, 248.9895)
  point P11 (-131, 229.0105)
  point P12 (-106, 242.4034)
  point P13 (-89.953, 251)
  point P14 (-122.047, 251)
  point P15 (-81, 50.9895)
  point P16 (-99.647, 41)
  point P17 (-81, 31.0105)
  point P18 (-131, 31.0105)
  point P19 (-112.353, 41)
  point P20 (-131, 50.9895)
  point P21 (-106, 44.4034)
  point P22 (-89.953, 53)
  point P23 (-122.047, 53)
  point P24 (-83.984, 98)
  point P25 (-106, 127.4857)
  point P26 (-128.016, 98)
  point P27 (-128.016, 167)
  point P28 (-106, 137.5143)
  point P29 (-83.984, 167)
  point P30 (-102.256, 132.5)
  point P31 (-81, 104.0322)
  point P32 (-81, 160.9678)
  point P33 (-131, 104.0322)
  point P34 (-109.744, 132.5)
  point P35 (-131, 160.9678)
  point P36 (-100.7506, 75.5)
  point P37 (-81, 61.7451)
  point P38 (-87.5571, 59)
  point P39 (-106, 71.8442)
  point P40 (-124.4429, 59)
  point P41 (-111.2494, 75.5)
  point P42 (-131, 89.2549)
  point P43 (-131, 61.7451)
  point P44 (-106, 79.1558)
  point P45 (-87.5571, 92)
  point P46 (-124.4429, 92)
  point P47 (-81, 177.0604)
  point P48 (-81, 216.9396)
  point P49 (-101.6781, 197)
  point P50 (-126.567, 173)
  point P51 (-85.433, 173)
  point P52 (-106, 192.8324)
  point P53 (-131, 177.0604)
  point P54 (-110.3219, 197)
  point P55 (-106, 201.1676)
  point P56 (-85.433, 221)
  point P57 (-126.567, 221)
  dimension "d290" = 3
  dimension "d291" = 3
  dimension "d292" = 3
  dimension "d293" = 3
  dimension "d294" = 3
  dimension "d295" = 3
  dimension "d296" = 3
  dimension "d297" = 3
  dimension "d298" = 3
  dimension "d299" = 3
  dimension "d300" = 3
  dimension "d301" = 3
  dimension "d302" = 3
  dimension "d303" = 3
  dimension "d304" = 3
  dimension "d305" = 3
  dimension "d306" = 3
  dimension "d307" = 3
  dimension "d308" = 3
  dimension "d309" = 3
  dimension "d310" = 3
  dimension "d311" = 3
  dimension "d320" = 3
  dimension "d321" = 3
  dimension "d322" = 3
  dimension "d323" = 3
  dimension "d324" = 3
  dimension "d325" = 3
  dimension "d326" = 3
  dimension "d327" = 3
  dimension "d328" = 3
  dimension "d329" = 3
  dimension "d330" = 3
  dimension "d331" = 3
  dimension "d332" = 3
  dimension "d333" = 3
  constraints: 140 end point, 32 parallel, 9 perpendicular, 2 midpoint, 2 vertical, 1 horizontal, 1 point on line, 8 other
  measures "d290" distance between parallel lines of L13 L18
  measures "d291" distance from line of L12 point (-131, 239)
  measures "d292" distance between parallel lines of L14 L25
  measures "d293" distance between parallel lines of L15 L23
  measures "d294" distance between parallel lines of L16 L24
  measures "d295" distance between parallel lines of L20 L16
  measures "d296" distance between parallel lines of L17 L19
  measures "d297" distance between parallel lines of L17 L22
  measures "d298" distance between parallel lines of L8 L26
  measures "d299" distance between parallel lines of L9 L28
  measures "d300" distance between parallel lines of L6 L29
  measures "d301" distance between parallel lines of L10 L32
  measures "d302" distance between parallel lines of L10 L30
  measures "d303" distance between parallel lines of L11 L33
  measures "d304" distance between parallel lines of L31 L11
  measures "d305" distance between parallel lines of L3 L34
  measures "d306" distance between parallel lines of L2 L42
  measures "d307" distance between parallel lines of L38 L2
  measures "d308" distance between parallel lines of L0 L35
  measures "d309" distance between parallel lines of L39 L0
  measures "d310" distance from line of L4 point (-131, 41)
  measures "d311" distance between parallel lines of L5 L37
  measures "d320" distance between parallel lines of L15 L51
  measures "d321" distance between parallel lines of L54 L50
  measures "d322" distance between parallel lines of L53 L50
  measures "d323" distance between parallel lines of L49 L56
  measures "d324" distance between parallel lines of L57 L49
  measures "d325" distance between parallel lines of L44 L60
  measures "d326" distance between parallel lines of L8 L58
  measures "d327" distance between parallel lines of L6 L61
  measures "d328" distance between parallel lines of L48 L65
  measures "d329" distance between parallel lines of L69 L48
  measures "d330" distance between parallel lines of L45 L62
  measures "d331" distance between parallel lines of L47 L66
  measures "d332" distance between parallel lines of L47 L64
  measures "d333" distance between parallel lines of L3 L68
extrude "押し出し27" cut sketch "スケッチ34" against normal blind 2 contours L34 L42 L35 | L64 L69 L68 | L62 L69 L66 | L39 L42 L41 | L38 L37 L35 | L64 L63 L65 | L65 L61 L66 | L28 L31 L32 | L30 L31 L29 | L33 L26 L32 | L30 L27 L33 | L52 L53 L56 | L57 L53 L58 | L51 L56 L54 | L57 L60 L54 | L22 L20 L21 | L24 L22 L23 | L18 L20 L19 | L24 L25 L19
sketch "スケッチ36" plane through (0, 0, -2) normal (0, 0, -1) x (-1, 0, 0)
  line L0 (-2, 285) -> (-188, 285) projected
  line L1 (-166.5226, 285) -> (-144, 285)
  line L2 (-144, 285) -> (-144, 15.7473)
  line L3 (-144, 15.7473) -> (-166.5226, 15.7473)
  line L4 (-166.5226, 15.7473) -> (-166.5226, 285)
  line L5 (-68, 285) -> (-20, 285)
  line L6 (-20, 285) -> (-20, 11.3003)
  line L7 (-20, 11.3003) -> (-68, 11.3003)
  line L8 (-68, 11.3003) -> (-68, 285)
  line L9 (-190, 5) -> (-190, 283) projected
  line L10 (0, 285) -> (-190, 285)
  line L11 (-190, 285) -> (-190, 265)
  line L12 (-190, 265) -> (0, 265)
  line L13 (0, 265) -> (0, 285)
  line L14 (0, 5) -> (0, 283) projected
  circle A0 centre (-78, 254) radius 3.75 projected
  circle A1 centre (-134, 254) radius 3.75 projected
  line L15 (-126.567, 173) -> (-106, 192.8324) projected
  line L16 (-106, 192.8324) -> (-85.433, 173) projected
  line L17 (-85.433, 173) -> (-126.567, 173) projected
  line L18 (-87.5571, 59) -> (-124.4429, 59) projected
  line L19 (-124.4429, 59) -> (-106, 71.8442) projected
  line L20 (-106, 71.8442) -> (-87.5571, 59) projected
  line L21 (-128.016, 167) -> (-83.984, 167) projected
  line L22 (-83.984, 167) -> (-106, 137.5143) projected
  line L23 (-106, 137.5143) -> (-128.016, 167) projected
  line L24 (-81, 50.9895) -> (-81, 31.0105) projected
  line L25 (-81, 31.0105) -> (-99.647, 41) projected
  line L26 (-99.647, 41) -> (-81, 50.9895) projected
  line L27 (-81, 229.0105) -> (-99.647, 239) projected
  line L28 (-99.647, 239) -> (-81, 248.9895) projected
  line L29 (-81, 248.9895) -> (-81, 229.0105) projected
  line L30 (-106, 242.4034) -> (-122.047, 251) projected
  line L31 (-122.047, 251) -> (-89.953, 251) projected
  line L32 (-89.953, 251) -> (-106, 242.4034) projected
  line L33 (-83.984, 98) -> (-128.016, 98) projected
  line L34 (-128.016, 98) -> (-106, 127.4857) projected
  line L35 (-106, 127.4857) -> (-83.984, 98) projected
  line L36 (-100.7506, 75.5) -> (-81, 89.2549) projected
  line L37 (-81, 89.2549) -> (-81, 61.7451) projected
  line L38 (-81, 61.7451) -> (-100.7506, 75.5) projected
  line L39 (-81, 177.0604) -> (-101.6781, 197) projected
  line L40 (-101.6781, 197) -> (-81, 216.9396) projected
  line L41 (-81, 216.9396) -> (-81, 177.0604) projected
  line L42 (-131, 177.0604) -> (-131, 216.9396) projected
  line L43 (-131, 216.9396) -> (-110.3219, 197) projected
  line L44 (-110.3219, 197) -> (-131, 177.0604) projected
  line L45 (-111.2494, 75.5) -> (-131, 61.7451) projected
  line L46 (-131, 61.7451) -> (-131, 89.2549) projected
  line L47 (-131, 89.2549) -> (-111.2494, 75.5) projected
  line L48 (-102.256, 132.5) -> (-81, 160.9678) projected
  line L49 (-81, 160.9678) -> (-81, 104.0322) projected
  line L50 (-81, 104.0322) -> (-102.256, 132.5) projected
  line L51 (-131, 31.0105) -> (-131, 50.9895) projected
  line L52 (-131, 50.9895) -> (-112.353, 41) projected
  line L53 (-112.353, 41) -> (-131, 31.0105) projected
  line L54 (-106, 235.5966) -> (-89.953, 227) projected
  line L55 (-89.953, 227) -> (-122.047, 227) projected
  line L56 (-122.047, 227) -> (-106, 235.5966) projected
  line L57 (-112.353, 239) -> (-131, 229.0105) projected
  line L58 (-131, 229.0105) -> (-131, 248.9895) projected
  line L59 (-131, 248.9895) -> (-112.353, 239) projected
  line L60 (-106, 44.4034) -> (-122.047, 53) projected
  line L61 (-122.047, 53) -> (-89.953, 53) projected
  line L62 (-89.953, 53) -> (-106, 44.4034) projected
  line L63 (-131, 104.0322) -> (-131, 160.9678) projected
  line L64 (-131, 160.9678) -> (-109.744, 132.5) projected
  line L65 (-109.744, 132.5) -> (-131, 104.0322) projected
  line L66 (-106, 79.1558) -> (-124.4429, 92) projected
  line L67 (-124.4429, 92) -> (-87.5571, 92) projected
  line L68 (-87.5571, 92) -> (-106, 79.1558) projected
  line L69 (-106, 201.1676) -> (-126.567, 221) projected
  line L70 (-126.567, 221) -> (-85.433, 221) projected
  line L71 (-85.433, 221) -> (-106, 201.1676) projected
  circle A2 centre (-180, 143) radius 3.75 projected
  circle A3 centre (-180, 243) radius 3.75 projected
  circle A4 centre (-180, 128) radius 3.75 projected
  circle A5 centre (-180, 258) radius 3.75 projected
  circle A6 centre (-180, 43) radius 3.75 projected
  arc A7 (-20, 5) -> (-18, 3) centre (-18, 5) ccw projected
  line L72 (-18, 3) -> (-2, 3) projected
  arc A8 (-2, 3) -> (0, 5) centre (-2, 5) ccw projected
  line L73 (0, 5) -> (0, 283) projected
  arc A9 (0, 283) -> (-2, 285) centre (-2, 283) ccw projected
  line L74 (-2, 285) -> (-188, 285) projected
  arc A10 (-188, 285) -> (-190, 283) centre (-188, 283) ccw projected
  line L75 (-190, 283) -> (-190, 22) projected
  arc A11 (-190, 22) -> (-188, 20) centre (-188, 22) ccw projected
  line L76 (-188, 20) -> (-187.1, 20) projected
  arc A12 (-187.1, 20) -> (-185.1, 22) centre (-187.1, 22) ccw projected
  line L77 (-185.1, 22) -> (-185.1, 28) projected
  arc A13 (-183.1, 30) -> (-185.1, 28) centre (-183.1, 28) ccw projected
  line L78 (-183.1, 30) -> (-161.9, 30) projected
  arc A14 (-159.9, 28) -> (-161.9, 30) centre (-161.9, 28) ccw projected
  line L79 (-159.9, 28) -> (-159.9, 22) projected
  arc A15 (-159.9, 22) -> (-157.9, 20) centre (-157.9, 22) ccw projected
  line L80 (-157.9, 20) -> (-113.1, 20) projected
  arc A16 (-113.1, 20) -> (-111.1, 22) centre (-113.1, 22) ccw projected
  line L81 (-111.1, 22) -> (-111.1, 28) projected
  arc A17 (-109.1, 30) -> (-111.1, 28) centre (-109.1, 28) ccw projected
  line L82 (-109.1, 30) -> (-87.9, 30) projected
  arc A18 (-85.9, 28) -> (-87.9, 30) centre (-87.9, 28) ccw projected
  line L83 (-85.9, 28) -> (-85.9, 22) projected
  arc A19 (-85.9, 22) -> (-83.9, 20) centre (-83.9, 22) ccw projected
  line L84 (-83.9, 20) -> (-22, 20) projected
  arc A20 (-20, 18) -> (-22, 20) centre (-22, 18) ccw projected
  line L85 (-20, 18) -> (-20, 5) projected
  circle A21 centre (-78, 26) radius 3.75 projected
  circle A22 centre (-78, 170) radius 3.75 projected
  circle A23 centre (-78, 254) radius 3.75 projected
  circle A24 centre (-134, 224) radius 3.75 projected
  circle A25 centre (-134, 95) radius 3.75 projected
  circle A26 centre (-134, 26) radius 3.75 projected
  circle A27 centre (-78, 56) radius 3.75 projected
  circle A28 centre (-134, 170) radius 3.75 projected
  circle A29 centre (-134, 254) radius 3.75 projected
  circle A30 centre (-78, 224) radius 3.75 projected
  circle A31 centre (-78, 95) radius 3.75 projected
  circle A32 centre (-134, 56) radius 3.75 projected
  point P0 (0, 0)
  point P1 (-155.2613, 285)
  point P2 (-20, 18)
  point P3 (-20, 265)
  point P4 (-68, 265)
  point P5 (-68, 20)
  point P6 (-144, 20)
  point P7 (-144, 265)
  point P8 (-166.5226, 265)
  point P9 (-166.5226, 30)
  dimension "d334" = 20
  dimension "d335" = 20
  dimension "d336" = 10
  dimension "d337" = 10
  constraints: 24 end point, 6 parallel, 4 point on line, 3 horizontal, 3 perpendicular, 1 midpoint
  measures "d334" distance from line of point (-155.261, 285) L12
  measures "d335" distance between parallel lines of L14 L6
  measures "d336" distance from line of A0.centre L8
  measures "d337" distance from line of A1.centre L2
extrude "押し出し28" cut sketch "スケッチ36" against normal blind 2 contours L6 A20 L84 L8 L12 | L2 L80 A15 L79 A14 L78 L4 L12
fillet "フィレット5" radius 2 7 edges at (166.5226, 30, -1) (144, 20, -1) (166.5226, 265, -1) (144, 265, -1) (68, 20, -1) (68, 265, -1) (20, 265, -1)
mirror "ミラー1" about plane through (0, 0, 0) normal (1, 0, 0)
sketch "スケッチ37" plane through (0, 0, 3) normal (0, 0, 1) x (1, 0, 0)
  line L0 (0, 315.7022) -> (241.7955, 315.7022)
  line L1 (241.7955, 315.7022) -> (241.7955, -25.5715)
  line L2 (241.7955, -25.5715) -> (0, -25.5715)
  line L3 (0, -25.5715) -> (0, 315.7022)
  point P0 (0, 0)
  constraints: 8 end point, 2 parallel, 1 horizontal, 1 perpendicular
extrude "押し出し29" cut sketch "スケッチ37" against normal blind 10
equation "\"d169\" = d168"
equation "\"d171\" = d167"
equation "\"d172\" = d171"
equation "\"d173\" = d168"
equation "\"d176\" = d175"
equation "\"d177\" = d171"
equation "\"d178\" = d171"
equation "\"d180\" = d179"
equation "\"d182\" = d181"
equation "\"d184\" = d183"
equation "\"d196\" = d195"
equation "\"d204\" = d193"
equation "\"d205\" = d195"
equation "\"d207\" = d205"
equation "\"d213\" = d212"
equation "\"d243\" = d242"
equation "\"d244\" = d242"
equation "\"d245\" = d242"
equation "\"d246\" = d244"
equation "\"d247\" = d245"
equation "\"d248\" = d246"
equation "\"d249\" = d247"
equation "\"d250\" = d248"
equation "\"d251\" = d249"
equation "\"d252\" = d250"
equation "\"d253\" = d251"
equation "\"d258\" = d257"
equation "\"d259\" = d256"
